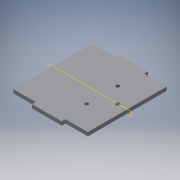
# Autodesk Inventor part: Pan base cross bar
Saved by Autodesk Inventor 2018 (Build 220112000, 112)
## iProperties
Created: 2018-06-25
Part Number: Pan base cross bar
Material: Generic
Document SubType Name: Modeling
Designer: Ajith Thomas
Density: 1 g/cm^3
Appearance: Default
Author: Ajith Thomas
Autodesk Inventor part; units mm, degrees
ref_plane "YZ Plane" through (0, 0, 0) normal (1, 0, 0) x (0, 1, 0)
ref_plane "XZ Plane" through (0, 0, 0) normal (0, 1, 0) x (-1, 0, 0)
ref_plane "XY Plane" through (0, 0, 0) normal (0, 0, 1) x (1, 0, 0)
sketch "Sketch1" plane through (0, 0, 0) normal (0, 0, 1) x (1, 0, 0)
  line L0 (2, -6) -> (2, -9) construction
  line L1 (-22, -9) -> (-22, -6) construction
  line L2 (20, -40) -> (20, -3) construction
  line L3 (-40, -3) -> (-40, -40) construction
  line L4 (20, -9) -> (-40, -9)
  line L5 (-40, -9) -> (-40, -6)
  line L6 (-40, -6) -> (20, -6)
  line L7 (20, -6) -> (20, -9)
  point P0 (0, 0)
  dimension "d0" = 3
  dimension "d1" = 60
  constraints: 8 end point, 2 parallel, 2 point on line, 1 horizontal, 1 perpendicular
  measures "d0" distance between parallel lines of L6 L4
  measures "d1" distance of L4.start L4.end
extrude "Extrusion1" add sketch "Sketch1" along normal blind 63.5
sketch "Sketch2" plane through (0, 0, 63.5) normal (0, 0, 1) x (1, 0, 0)
  line L0 (-22, -9) -> (-22, -6) projected
  line L1 (2, -9) -> (-22, -9) projected
  line L2 (-22, -6) -> (2, -6) projected
  line L3 (2, -6) -> (2, -9) projected
  point P0 (0, 0)
extrude "Extrusion2" add sketch "Sketch2" along normal blind 3
ref_plane "Work Plane1" through (0, 0, 31.75) normal (0, 0, 1) x (1, 0, 0)
mirror "Mirror1" about plane through (0, 0, 31.75) normal (0, 0, 1) of "Extrusion2"
sketch "Sketch3" plane through (20, -9, 0) normal (0, -1, 0) x (1, 0, 0)
  circle A0 centre (-7.5, 31.75) radius 1.5 projected
  circle A1 centre (-20, 44.25) radius 1.5 projected
  circle A2 centre (-20, 19.25) radius 1.5 projected
  point P0 (-20, 0)
extrude "Extrusion3" cut sketch "Sketch3" against normal blind 3
body "Solid1"
